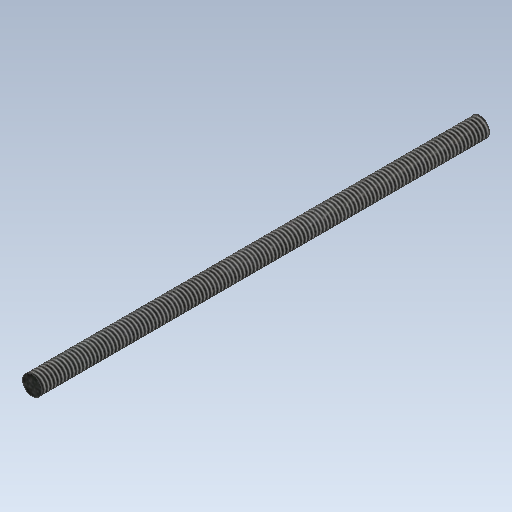
# Autodesk Inventor part: 0008-10-1003 T8 screw
Saved by Autodesk Inventor 2020 (Build 240168000, 168)
## iProperties
Created: 2021-02-20
Part Number: 0008-10-1003 T8 screw
Material: Steel
Document SubType Name: Modeling
Designer: Iulian Bors
Density: 7.85 g/cm^3
Appearance: Plate
Mass: 69.0522 g
Surface Area: 44.9876 cm^2
Volume: 8.79646 cm^3
Description: Surub T8
d0: 8.000 mm
d1: 185.000 mm
Author: Iulian Bors
Subject: 1003
Autodesk Inventor part; units mm, degrees
ref_plane "YZ Plane" through (0, 0, 0) normal (1, 0, 0) x (0, 1, 0)
ref_plane "XZ Plane" through (0, 0, 0) normal (0, 1, 0) x (-1, 0, 0)
ref_plane "XY Plane" through (0, 0, 0) normal (0, 0, 1) x (1, 0, 0)
sketch "Sketch1" plane through (0, 0, 0) normal (0, 0, 1) x (1, 0, 0)
  circle A0 centre (0.2231, 0) radius 4
  point P0 (0, 0)
  dimension "d0" = 8
  constraints: 1 centre point
  measures "d0" diameter of A0
extrude "Extrusion1" add sketch "Sketch1" along normal blind 185
thread "Thread1" size "TR8x1.5" class "7e" standard "ISO Metric Trapezoidal Threads" full length
body "Solid1"
